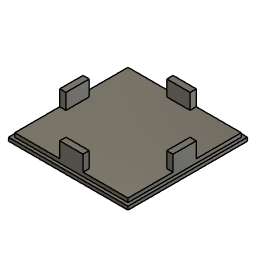
caja  modulos y sensores v4 (Autodesk Fusion 360 design; units mm, degrees)
Autodesk Fusion 360 part; units mm, degrees
sketch "Sketch1" plane through (0, 0, 0) normal (0, 1, 0) x (1, 0, 0)
  line L0 (-125.1981, 84.6119) -> (24.8019, 84.6119)
  line L1 (24.8019, 84.6119) -> (24.8019, -65.3881)
  line L2 (24.8019, -65.3881) -> (-125.1981, -65.3881)
  line L3 (-125.1981, -65.3881) -> (-125.1981, 84.6119)
  dimension "d1" = 150
  dimension "d2" = 150
  constraint horizontal L0
  constraint vertical L1
  constraint horizontal L2
  constraint vertical L3
  measures "d1" distance of L0.start L0.end
  measures "d2" distance of L0.start L2.end
extrude "Extrude1" add sketch "Sketch1" along normal blind 50 makes body 1
shell "Shell1" thickness 0.2 outward thickness 2 removed faces 1 at (-75.1981, 50, -34.6119) on bodies 1
sketch "Sketch2" plane through (0, 0, 0) normal (0, 1, 0) x (1, 0, 0)
  line L0 (63.7249, 81.3624) -> (217.7249, 81.3624)
  line L1 (217.7249, 81.3624) -> (217.7249, -72.6376)
  line L2 (217.7249, -72.6376) -> (63.7249, -72.6376)
  line L3 (63.7249, -72.6376) -> (63.7249, 81.3624)
  dimension "d7" = 154
  dimension "d8" = 154
  constraint horizontal L0
  constraint vertical L1
  constraint horizontal L2
  constraint vertical L3
  measures "d7" distance of L0.start L0.end
  measures "d8" distance of L0.start L2.end
extrude "Extrude2" add sketch "Sketch2" along normal blind 4 separate body makes body 2
sketch "Sketch3" plane through (0, 4, 0) normal (0, 1, 0) x (-1, 0, 0)
  line L0 (-63.7249, 72.6376) -> (-217.7249, 72.6376)
  line L1 (-217.7249, 72.6376) -> (-217.7249, -81.3624)
  line L2 (-217.7249, -81.3624) -> (-63.7249, -81.3624)
  line L3 (-63.7249, -81.3624) -> (-63.7249, 72.6376)
  line L4 (-67.7249, -77.3624) -> (-67.7249, 68.6376)
  line L5 (-213.7249, -77.3624) -> (-213.7249, 68.6376)
  line L6 (-140.7249, -77.3624) -> (-67.7249, -77.3624)
  line L7 (-140.7249, -77.3624) -> (-213.7249, -77.3624)
  line L8 (-140.7249, 68.6376) -> (-213.7249, 68.6376)
  line L9 (-140.7249, 68.6376) -> (-67.7249, 68.6376)
extrude "Extrude3" add sketch "Sketch3" along normal blind 5 contours L4 L5 L6 L7 L8 L9 bodies 2
sketch "Sketch4" plane through (0, 9, 0) normal (0, 1, 0) x (-1, 0, 0)
  line L0 (-213.7249, -77.3624) -> (-67.7249, -77.3624)
  line L1 (-67.7249, -77.3624) -> (-67.7249, 68.6376)
  line L2 (-67.7249, 68.6376) -> (-213.7249, 68.6376)
  line L3 (-213.7249, 68.6376) -> (-213.7249, -77.3624)
  line L4 (-125.7249, -77.3624) -> (-155.7249, -77.3624)
  line L5 (-155.7249, -77.3624) -> (-155.7249, -69.3624)
  line L6 (-155.7249, -69.3624) -> (-125.7249, -69.3624)
  line L7 (-125.7249, -69.3624) -> (-125.7249, -77.3624)
  line L8 (-155.7249, 60.6376) -> (-125.7249, 60.6376)
  line L9 (-155.7249, -77.3624) -> (-155.7249, -69.3624)
  line L10 (-125.7249, -77.3624) -> (-125.7249, -69.3624)
  line L11 (-125.7249, 60.6376) -> (-125.7249, 68.6376)
  line L12 (-155.7249, 60.6376) -> (-155.7249, 68.6376)
  line L13 (-67.7249, -19.3624) -> (-75.7249, -19.3624)
  line L14 (-75.7249, -19.3624) -> (-75.7249, 10.6376)
  line L15 (-75.7249, 10.6376) -> (-67.7249, 10.6376)
  line L16 (-67.7249, 10.6376) -> (-67.7249, -19.3624)
  line L17 (-75.7249, -19.3624) -> (-67.7249, -19.3624)
  line L18 (-75.7249, 10.6376) -> (-67.7249, 10.6376)
  line L19 (-205.7249, -19.3624) -> (-205.7249, 10.6376)
  line L20 (-205.7249, -19.3624) -> (-213.7249, -19.3624)
  line L21 (-213.7249, 10.6376) -> (-213.7249, -19.3624)
  line L22 (-205.7249, 10.6376) -> (-213.7249, 10.6376)
  dimension "d18" = 8
  dimension "d19" = 8
  constraint horizontal L4
  constraint vertical L5
  constraint horizontal L6
  constraint vertical L7
  constraint horizontal L13
  constraint vertical L14
  constraint horizontal L15
  constraint vertical L16
  measures "d18" distance of L4.start L6.end
  measures "d19" distance of L13.start L13.end
extrude "Extrude4" add sketch "Sketch4" along normal blind 20 contours L0 L4 L5 L6 L7 L9 L10 | L3 L19 L20 L21 L22 | L1 L13 L14 L15 L16 L17 L18 | L2 L8 L11 L12 bodies 2
move_face "OffsetFaces1" offset 0.4 1 faces at (115.0582, 0, -30.0291) on bodies 2
hidden bodies 1
